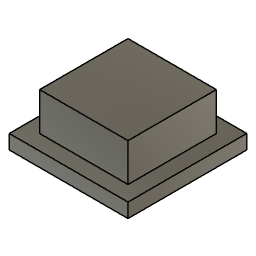
button-cap v2 (Autodesk Fusion 360 design; units mm, degrees)
Autodesk Fusion 360 part; units mm, degrees
sketch "Sketch1" plane through (0, 0, 0) normal (0, 0, 1) x (1, 0, 0)
  line L0 (0, 0) -> (6.5, 0)
  line L1 (6.5, 0) -> (6.5, 6.5)
  line L2 (6.5, 6.5) -> (0, 6.5)
  line L3 (0, 6.5) -> (0, 0)
  line L4 (0, 3.25) -> (6.5, 3.25) construction
  line L5 (3.25, 6.5) -> (3.25, 0) construction
  circle A0 centre (3.25, 3.25) radius 1.75
  line L6 (-1.4, 7.9) -> (-1.4, -1.4)
  line L7 (-1.4, -1.4) -> (7.9, -1.4)
  line L8 (7.9, -1.4) -> (7.9, 7.9)
  line L9 (7.9, 7.9) -> (-1.4, 7.9)
  line L10 (-3, 9.5) -> (-3, -3)
  line L11 (-3, -3) -> (9.5, -3)
  line L12 (9.5, -3) -> (9.5, 9.5)
  line L13 (9.5, 9.5) -> (-3, 9.5)
  dimension "d1" = 6.5
  dimension "d2" = 6.5
  dimension "d3" = 3.5
  dimension "d4" = 1.4
  dimension "d5" = 3
  constraint horizontal L0
  constraint vertical L1
  constraint horizontal L2
  constraint vertical L3
  constraint coincident L0.start L3.end
  constraint midpoint L3 L4.start
  constraint midpoint L1 L4.end
  constraint midpoint L2 L5.start
  constraint midpoint L0 L5.end
  constraint midpoint L4 A0.centre
  measures "d1" distance of L0.start L0.end
  measures "d2" distance of L0.start L2.end
  measures "d3" diameter of A0
extrude "Extrude1" add sketch "Sketch1" along normal blind 7 contours L6 L7 L8 L9
extrude "Extrude2" add sketch "Sketch1" along normal blind 1.5 from surface at 1.5 contours L10 L11 L12 L13
extrude "Extrude3" add sketch "Sketch1" along normal blind 3.5 from surface at 3.5 contours L0 L1 L2 L3 | A0
extrude "Extrude4" cut sketch "Sketch1" along normal blind 4 contours A0
